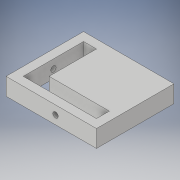
# Autodesk Inventor part: odometery system base
Saved by Autodesk Inventor 2019 (Build 230136000, 136)
## iProperties
Created: 2019-08-10
Part Number: odometery system base
Material: Generic
Document SubType Name: Modeling
Designer: Delta
Density: 1 g/cm^3
Appearance: Default
Author: Delta
Autodesk Inventor part; units mm, degrees
ref_plane "YZ Plane" through (0, 0, 0) normal (1, 0, 0) x (0, 1, 0)
ref_plane "XZ Plane" through (0, 0, 0) normal (0, 1, 0) x (-1, 0, 0)
ref_plane "XY Plane" through (0, 0, 0) normal (0, 0, 1) x (1, 0, 0)
sketch "Sketch1" plane through (0, 0, 0) normal (0, 1, 0) x (-1, 0, 0)
  line L0 (0, 0) -> (133.35, 0)
  line L1 (133.35, 0) -> (133.35, 114.3)
  line L2 (133.35, 114.3) -> (0, 114.3)
  line L3 (0, 114.3) -> (0, 0)
  line L4 (12.7, 12.7) -> (120.65, 12.7)
  line L5 (120.65, 12.7) -> (120.65, 101.6)
  line L6 (120.65, 101.6) -> (12.7, 101.6)
  line L7 (12.7, 101.6) -> (12.7, 12.7)
  line L8 (12.7, 12.7) -> (101.6, 12.7)
  line L9 (101.6, 12.7) -> (101.6, 82.55)
  line L10 (101.6, 82.55) -> (12.7, 82.55)
  line L11 (12.7, 82.55) -> (12.7, 12.7)
  dimension "d0" = 114.3
  dimension "d1" = 133.35
  dimension "d2" = 12.7
  dimension "d3" = 12.7
  dimension "d4" = 12.7
  dimension "d5" = 12.7
  dimension "d6" = 19.05
  dimension "d7" = 19.05
  constraints: 24 end point, 6 parallel, 3 horizontal, 3 perpendicular
  measures "d0" distance of L1.end L0.end
  measures "d1" distance of L2.end L1.end
  measures "d2" distance between parallel lines of L0 L4
  measures "d3" distance between parallel lines of L2 L6
  measures "d4" distance between parallel lines of L1 L5
  measures "d5" distance between parallel lines of L3 L7
  measures "d6" distance between parallel lines of L6 L10
  measures "d7" distance between parallel lines of L5 L9
extrude "Extrusion1" add sketch "Sketch1" along normal blind 25.4 contours L3 L2 L1 L0 | L7 L10 L9 L4
sketch "Sketch3" plane through (-133.35, 0, 114.3) normal (0, 0, 1) x (1, 0, 0)
  line L0 (133.35, 0) -> (133.35, 25.4) projected
  line L1 (0, 25.4) -> (133.35, 25.4) projected
  line L2 (12.7, 0) -> (12.7, 25.4) projected
  point P0 (73.025, 12.7)
  dimension "d10" = 120.65
  dimension "d11" = 25.4
  dimension "d12" = 60.325
  dimension "d13" = 12.7
  measures "d10" distance between parallel lines of L2 L0
  measures "d11" distance of L0.start L0.end
  measures "d12" distance from line of L0 point (73.025, 12.7)
  measures "d13" distance from line of L1 point (73.025, 12.7)
hole "Hole1" at (-60.325, 12.7, 114.3) direction (0, 0, -1) diameter 7.85 depth 12.7 tip angle 118
sketch "Sketch4" plane through (-133.35, 0, 0) normal (-1, 0, 0) x (0, 0, 1)
  line L0 (0, 25.4) -> (114.3, 25.4) projected
  line L1 (114.3, 0) -> (114.3, 25.4) projected
  point P0 (0, 0)
  point P1 (57.15, 12.7)
  dimension "d21" = 25.4
  dimension "d22" = 114.3
  dimension "d23" = 12.7
  dimension "d24" = 57.15
  measures "d21" distance of L1.start L0.end
  measures "d22" distance of L0.start L0.end
  measures "d23" distance from line of L0 point (57.15, 12.7)
  measures "d24" distance from line of L1 point (57.15, 12.7)
hole "Hole2" at (-133.35, 12.7, 57.15) direction (1, 0, 0) diameter 7.85 depth 12.7
equation "\"d3\" = d2"
equation "\"d4\" = d2"
equation "\"d5\" = d2"
equation "\"d6\" = d7"
equation "\"d12\" = 0.5 * d10"
equation "\"d13\" = 0.5 * d11"
equation "\"d23\" = 0.5 * d21"
equation "\"d24\" = 0.5 * d22"
body "Solid1"
